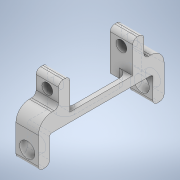
# Autodesk Inventor part: 14mmto28mm
Saved by Autodesk Inventor 2020.2 (Build 242310000, 310)
## iProperties
Created: 2025-05-27
Part Number: 14mmto28mm
Material: Типовые
Document SubType Name: Modeling
Designer: Кир
Density: 1 g/cm^3
Appearance: По умолчанию
Author: Кир
Autodesk Inventor part; units mm, degrees
ref_plane "YZ Plane" through (0, 0, 0) normal (1, 0, 0) x (0, 1, 0)
ref_plane "XZ Plane" through (0, 0, 0) normal (0, 1, 0) x (-1, 0, 0)
ref_plane "XY Plane" through (0, 0, 0) normal (0, 0, 1) x (1, 0, 0)
sketch "Эскиз1" plane through (0, 0, 0) normal (0, 1, 0) x (-1, 0, 0)
  line L0 (-7, -7) -> (7, -7)
  line L1 (7, -7) -> (7, 7)
  line L2 (7, 7) -> (-7, 7)
  line L3 (-7, 7) -> (-7, -7)
  line L4 (-7, -7) -> (7, 7) construction
  line L5 (7, -7) -> (-7, 7) construction
  line L6 (-14, -14) -> (14, -14)
  line L7 (14, -14) -> (14, 14)
  line L8 (14, 14) -> (-14, 14)
  line L9 (-14, 14) -> (-14, -14)
  line L10 (-14, -14) -> (14, 14) construction
  line L11 (14, -14) -> (-14, 14) construction
  point P0 (0, 0)
  dimension "d0" = 14
  dimension "d1" = 14
  dimension "d2" = 28
  dimension "d3" = 28
  constraints: 24 end point, 4 midpoint, 4 parallel, 2 horizontal, 2 perpendicular
  measures "d0" distance of L2.end L1.end
  measures "d1" distance of L1.end L0.end
  measures "d2" distance of L8.end L7.end
  measures "d3" distance of L7.end L6.end
extrude "Выдавливание1" add sketch "Эскиз1" along normal blind 15
sketch "Эскиз2" plane through (0, 15, 0) normal (0, 1, 0) x (1, 0, 0)
  line L0 (9.5, 9.5) -> (-9.5, 9.5)
  line L1 (-9.5, 9.5) -> (-9.5, -9.5)
  line L2 (-9.5, -9.5) -> (9.5, -9.5)
  line L3 (9.5, -9.5) -> (9.5, 9.5)
  line L4 (9.5, 9.5) -> (-9.5, -9.5) construction
  line L5 (-9.5, 9.5) -> (9.5, -9.5) construction
  line L6 (-14, 14) -> (-14, -14) projected
  line L7 (14, 14) -> (-14, 14)
  line L8 (-14, 14) -> (-14, -14)
  line L9 (-14, -14) -> (14, -14)
  line L10 (14, -14) -> (14, 14)
  line L11 (14, 14) -> (-14, -14) construction
  line L12 (-14, 14) -> (14, -14) construction
  point P0 (0, 0)
  dimension "d6" = 19
  dimension "d7" = 19
  constraints: 24 end point, 4 midpoint, 4 parallel, 2 horizontal, 2 perpendicular
  measures "d6" distance of L2.end L1.end
  measures "d7" distance of L1.end L0.end
extrude "Выдавливание2" cut sketch "Эскиз2" against normal blind 5
sketch "Эскиз4" plane through (-9.5, 15, 9.5) normal (0, 0, 1) x (1, 0, 0)
  point P0 (9.5, -15)
  point P1 (9.5, -2.5)
hole "Отверстие1" at (0, 12.5, 9.5) direction (0, 0, -1) diameter 2.4 end through all clearance for "Винт крепежный с плоской головкой" size "M2" standard "ANSI метрическая"
sketch "Эскиз5" plane through (-14, 0, 14) normal (0, 0, 1) x (1, 0, 0)
  point P0 (14, 0)
  point P1 (14.0165, 2.9909)
hole "Отверстие2" at (0.0165, 2.9909, 14) direction (0, 0, -1) diameter 3.4 end through all clearance for "Винт крепежный с плоской головкой" size "M3" standard "ANSI метрическая"
sketch "Эскиз6" plane through (0, 0, 0) normal (0, -1, 0) x (1, 0, 0)
  line L0 (11.5, -11.5) -> (-11.5, -11.5)
  line L1 (-11.5, -11.5) -> (-11.5, 11.5)
  line L2 (-11.5, 11.5) -> (11.5, 11.5)
  line L3 (11.5, 11.5) -> (11.5, -11.5)
  line L4 (11.5, -11.5) -> (-11.5, 11.5) construction
  line L5 (-11.5, -11.5) -> (11.5, 11.5) construction
  point P0 (0, 0)
  dimension "d24" = 23
  dimension "d25" = 23
  constraints: 12 end point, 2 midpoint, 2 parallel, 1 horizontal, 1 perpendicular
  measures "d24" distance of L1.end L2.end
  measures "d25" distance of L0.end L1.end
extrude "Выдавливание3" cut sketch "Эскиз6" against normal blind 6
sketch "Эскиз7" plane through (-14, 0, -14) normal (-1, 0, 0) x (0, 0, 1)
  line L0 (28, 0) -> (28, 10) projected
  line L1 (28, 0) -> (0, 0)
  line L2 (0, 0) -> (0, 15.2302)
  line L3 (0, 15.2302) -> (28, 15.2302)
  line L4 (28, 15.2302) -> (28, 0)
  point P0 (14, 0)
  constraints: 8 end point, 2 parallel, 1 horizontal, 1 perpendicular
extrude "Выдавливание4" cut sketch "Эскиз7" against normal blind 11.5
sketch "Эскиз8" plane through (14, 0, 14) normal (1, 0, 0) x (0, 0, -1)
  line L0 (0, 0) -> (28, 0) projected
  line L1 (28, 0) -> (0, 0)
  line L2 (0, 0) -> (0, 16.0654)
  line L3 (0, 16.0654) -> (28, 16.0654)
  line L4 (28, 16.0654) -> (28, 0)
  point P0 (14, 0)
  constraints: 8 end point, 2 parallel, 1 horizontal, 1 perpendicular
extrude "Выдавливание5" cut sketch "Эскиз8" against normal blind 11.5
sketch "Эскиз9" plane through (-2.5, 6, 7) normal (0, 0, -1) x (-1, 0, 0)
  line L0 (-5, 9) -> (-5, 0) projected
  line L1 (-5, 0) -> (-4, 0)
  line L2 (-4, 0) -> (-4, 2)
  line L3 (-4, 2) -> (-5, 2)
  line L4 (-5, 2) -> (-5, 0)
  point P0 (-2.5, -6)
  dimension "d32" = 1
  dimension "d35" = 2
  constraints: 8 end point, 2 parallel, 1 horizontal, 1 perpendicular
  measures "d32" distance of L3.end L2.end
  measures "d35" distance between parallel lines of L1 L3
extrude "Выдавливание6" add sketch "Эскиз9" along normal blind 14
fillet "Сопряжение1" radius 2 2 edges at (1.5, 7, 7) (1.5, 7, -7)
fillet "Сопряжение1" radius 1 10 edges at (0, 15, 9.5) (0, 15, 7) (0, 15, -9.5) (0, 15, -7) (0, 10, -9.5) (0, 10, 9.5) (0, 0, 11.5) (0, 0, 14) (0, 0, -14) (0, 0, -11.5)
fillet "Сопряжение1" radius 0.5 2 edges at (0, 6, 11.5) (0, 6, -11.5)
fillet "Сопряжение1" radius 3 2 edges at (0, 10, -14) (0, 10, 14)
